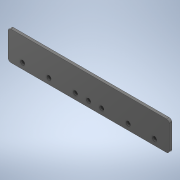
# Autodesk Inventor part: line_sensor
Saved by Autodesk Inventor 2020 (Build 240168000, 168)
## iProperties
Created: 2020-06-24
Part Number: line_sensor
Material: アセタール樹脂、黒
Document SubType Name: Modeling
Designer: haya
Density: 1.425 g/cm^3
Appearance: 滑らか - 黒
Author: haya
Autodesk Inventor part; units mm, degrees
ref_plane "YZ Plane" through (0, 0, 0) normal (1, 0, 0) x (0, 1, 0)
ref_plane "XZ Plane" through (0, 0, 0) normal (0, 1, 0) x (-1, 0, 0)
ref_plane "XY Plane" through (0, 0, 0) normal (0, 0, 1) x (1, 0, 0)
sketch "スケッチ1" plane through (0, 0, 0) normal (0, 0, 1) x (1, 0, 0)
  line L0 (0, 0) -> (122, 0)
  line L1 (122, 0) -> (122, 22)
  line L2 (122, 22) -> (0, 22)
  line L3 (0, 22) -> (0, 0)
  dimension "d0" = 122
  dimension "d1" = 22
  constraints: 8 end point, 2 parallel, 1 horizontal, 1 perpendicular
  measures "d0" distance of L0.start L0.end
  measures "d1" distance of L2.end L0.start
extrude "押し出し1" add sketch "スケッチ1" along normal blind 2
fillet "フィレット1" radius 2 4 edges at (122, 22, 1) (122, 0, 1) (0, 22, 1) (0, 0, 1)
sketch "スケッチ2" plane through (0, 0, 2) normal (0, 0, 1) x (1, 0, 0)
  line L0 (0, 4.5) -> (122, 4.5)
  line L1 (122, 2) -> (122, 20) projected
  line L2 (2, 0) -> (120, 0) projected
  line L3 (0, 20) -> (0, 2) projected
  point P0 (0, 0)
  point P1 (11, 4.5)
  point P2 (31, 4.5)
  point P3 (51, 4.5)
  point P4 (61, 4.5)
  point P5 (71, 4.5)
  point P6 (91, 4.5)
  point P7 (111, 4.5)
  dimension "d5" = 4.5
  dimension "d6" = 11
  dimension "d7" = 11
  dimension "d8" = 20
  dimension "d9" = 20
  dimension "d10" = 10
  dimension "d11" = 10
  dimension "d12" = 20
  constraints: 1 point on line, 10 other
  measures "d6" distance from line of point (11, 4.5) L3
  measures "d7" distance from line of point (111, 4.5) L1
  measures "d8" distance of point (111, 4.5) point (91, 4.5)
  measures "d9" distance of point (91, 4.5) point (71, 4.5)
  measures "d10" distance of point (71, 4.5) point (61, 4.5)
  measures "d11" distance of point (61, 4.5) point (51, 4.5)
  measures "d12" distance of point (51, 4.5) point (31, 4.5)
hole "穴1" at (11, 4.5, 2) at (31, 4.5, 2) at (51, 4.5, 2) at (61, 4.5, 2) at (71, 4.5, 2) at (91, 4.5, 2) at (111, 4.5, 2) direction (0, 0, -1) diameter 3.2 end through all
